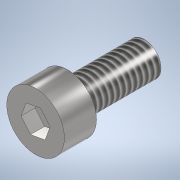
# Autodesk Inventor part: ネジキャップM2.6L6ステンレス
Saved by Autodesk Inventor 2020.2 (Build 242310000, 310)
## iProperties
Created: 2020-04-15
Part Number: ネジキャップM2.6L6ステンレス
Material: ステンレス鋼
Document SubType Name: Modeling
Designer: aoyama
Density: 8 g/cm^3
Appearance: 半つや出し
Author: aoyama
Autodesk Inventor part; units mm, degrees
ref_plane "YZ Plane" through (0, 0, 0) normal (1, 0, 0) x (0, 1, 0)
ref_plane "XZ Plane" through (0, 0, 0) normal (0, 1, 0) x (-1, 0, 0)
ref_plane "XY Plane" through (0, 0, 0) normal (0, 0, 1) x (1, 0, 0)
sketch "スケッチ1" plane through (0, 0, 0) normal (0, 0, 1) x (1, 0, 0)
  circle A0 centre (0, 0) radius 2.25
  circle A1 centre (0, 0) radius 1.3
  dimension "d0" = 4.5
  dimension "d6" = 2.6
  constraints: 2 centre point, 2 coincident
  measures "d0" diameter of A0
  measures "d6" diameter of A1
extrude "押し出し1" add sketch "スケッチ1" along normal blind 2.5 contours A0 | A1
sketch "スケッチ2" plane through (0, 0, 2.5) normal (0, 0, 1) x (1, 0, 0)
  circle A0 centre (0, 0) radius 2.25 projected
  line L0 (-0.3947, -1.0851) -> (-1.1371, -0.2007)
  line L1 (-1.1371, -0.2007) -> (-0.7424, 0.8844)
  line L2 (-0.7424, 0.8844) -> (0.3947, 1.0851)
  line L3 (0.3947, 1.0851) -> (1.1371, 0.2007)
  line L4 (1.1371, 0.2007) -> (0.7424, -0.8844)
  line L5 (0.7424, -0.8844) -> (-0.3947, -1.0851)
  dimension "d3" = 2
  constraints: 12 end point, 1 coincident, 13 other
  measures "d3" distance between parallel lines of L5 L2
extrude "押し出し2" cut sketch "スケッチ2" against normal blind 1.1 contours L0 L1 L2 L3 L4 L5
extrude "押し出し3" add sketch "スケッチ1" against normal blind 6 contours A1
thread "ねじ1" size "M2.6x0.45" class "6g" standard "ANSI Metric M Profile" length 44.8
